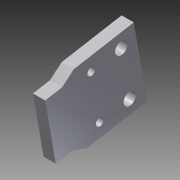
# Autodesk Inventor part: Arm_Link_1
Saved by Autodesk Inventor 2013 (Build 170138000, 138)
## iProperties
Created: 2014-05-15
Part Number: Arm_Link_1
Material: アセタール樹脂、白
Document SubType Name: Modeling
Designer: andou
Density: 1.425 g/cm^3
Mass: 3.20612 g
Surface Area: 16.6832 cm^2
Volume: 2.24991 cm^3
Author: andou
Autodesk Inventor part; units mm, degrees
ref_plane "YZ Plane" through (0, 0, 0) normal (1, 0, 0) x (0, 1, 0)
ref_plane "XZ Plane" through (0, 0, 0) normal (0, 1, 0) x (-1, 0, 0)
ref_plane "XY Plane" through (0, 0, 0) normal (0, 0, 1) x (1, 0, 0)
sketch "スケッチ2" plane through (0, 0, 0) normal (1, 0, 0) x (0, 1, 0)
  line L0 (0, 0) -> (-84.4498, 0)
  line L1 (-84.4498, -20) -> (1.7498, -20)
  line L2 (0, 0) -> (83.1668, 14.6646)
  line L3 (86.6398, -5.0316) -> (1.7498, -20)
  arc A0 (87.251, 14.537) -> (83.1668, 14.6646) centre (84.9033, 4.8165) ccw
  arc A1 (86.6398, -5.0316) -> (90.434, -3.5148) centre (84.9033, 4.8165) ccw
  arc A2 (-88.4498, -19.1652) -> (-84.4498, -20) centre (-84.4498, -10) ccw
  arc A3 (-84.4498, 0) -> (-88.4498, -0.8348) centre (-84.4498, -10) ccw
  arc A4 (-84.4498, -14) -> (-84.4498, -6) centre (-84.4498, -10) ccw
  line L4 (-84.4498, -6) -> (-88.4498, -6)
  line L5 (-84.4498, -14) -> (-88.4498, -14)
  line L6 (-88.4498, -0.8348) -> (-88.4498, -6)
  line L7 (-88.4498, -14) -> (-88.4498, -19.1652)
  line L8 (87.251, 14.537) -> (88.1479, 9.4503)
  line L9 (89.5371, 1.5718) -> (90.434, -3.5148)
  line L10 (1.7498, -20) -> (0, 0)
  line L11 (88.1479, 9.4503) -> (89.5371, 1.5718)
  dimension "d21" = 20
  dimension "d22" = 10
  dimension "d23" = 170
  dimension "d25" = 10
  dimension "d27" = 10
  dimension "d31" = 8
  dimension "d33" = 4
  dimension "d35" = 4
  dimension "d36" = 170
  constraints: 24 end point, 10 point on circle, 8 perpendicular, 5 centre point, 4 equal length, 3 equal radius, 2 parallel, 2 tangent, 1 coincident, 1 collinear, 1 horizontal
  measures "d21" distance between parallel lines of L0 L1
  measures "d22" distance from line of L0 A2.centre
  measures "d23" angle of L0 L2
  measures "d25" distance from line of L3 A0.centre
  measures "d27" radius of A3
  measures "d31" diameter of A4
  measures "d33" distance from line of L6 A2.centre
  measures "d35" distance from line of L8 L2.end
  measures "d36" distance of A2.centre A0.centre
extrude "押し出し1" add sketch "スケッチ2" along normal blind 4
sketch "スケッチ4" plane through (0, 0, 0) normal (-1, 0, 0) x (0, 0, 1)
  line L0 (-20, 1.7498) -> (-5.0316, 86.6398) projected
  line L1 (-20, -84.4498) -> (-20, 1.7498) projected
  circle A0 centre (-15, -8.7259) radius 1
  circle A1 centre (-13.2569, 11.198) radius 1
  line L2 (-15, -8.7259) -> (-13.2569, 11.198)
  dimension "d57" = 2
  dimension "d59" = 20
  dimension "d60" = 175
  dimension "d61" = 5
  dimension "d62" = 5
  constraints: 2 centre point, 2 end point, 1 equal radius
  measures "d57" diameter of A0
  measures "d59" distance of L2.start L2.end
  measures "d60" angle of L1 L2
  measures "d61" distance from line of L1 L2.start
  measures "d62" distance from line of L0 L2.end
hole "穴2" at (0, -8.7259, -15) at (0, 11.198, -13.2569) direction (1, 0, 0) diameter 1.6 end through all
sketch "スケッチ6" plane through (4, 0, 0) normal (1, 0, 0) x (0, 0, -1)
  line L0 (20, 1.7498) -> (5.0316, 86.6398) projected
  arc A0 (5.0316, 86.6398) -> (3.5148, 90.434) centre (-4.8165, 84.9033) ccw projected
  line L1 (3.5148, 90.434) -> (-14.537, 87.251) projected
  arc A1 (-14.537, 87.251) -> (-14.6646, 83.1668) centre (-4.8165, 84.9033) ccw projected
  line L2 (-14.6646, 83.1668) -> (0, 0) projected
  line L3 (-9.3978, 53.2975) -> (-12.6117, 57.1277)
  line L4 (-14.537, 87.251) -> (-17.8212, 86.6719)
  line L5 (-17.8212, 86.6719) -> (-12.6117, 57.1277)
  line L6 (3.5148, 90.434) -> (6.799, 91.0131)
  line L7 (6.799, 91.0131) -> (12.0085, 61.4689)
  line L8 (12.0085, 61.4689) -> (10.2984, 56.7704)
  dimension "d75" = 150
  dimension "d76" = 150
  dimension "d77" = 2.5
  dimension "d78" = 2.5
  dimension "d79" = 30
  constraints: 12 end point, 3 parallel, 2 collinear, 2 point on line
  measures "d75" angle of L2 L3
  measures "d76" angle of L0 L8
  measures "d77" distance between parallel lines of L0 L7
  measures "d78" distance between parallel lines of L2 L5
  measures "d79" distance of L4.end L3.end
extrude "押し出し2" add sketch "スケッチ6" against normal blind 4
sketch "スケッチ5" plane through (4, 0, 0) normal (1, 0, 0) x (0, 0, -1)
  line L0 (3.5148, 90.434) -> (-14.537, 87.251) projected
  line L1 (-14.6646, 83.1668) -> (0, 0) projected
  circle A0 centre (-10.7848, 72.6812) radius 1.5
  circle A1 centre (4.9721, 75.4596) radius 1.5
  line L2 (-12.6117, 57.1277) -> (-17.8212, 86.6719) projected
  line L3 (-17.8212, 86.6719) -> (6.799, 91.0131) projected
  line L4 (6.799, 91.0131) -> (12.0085, 61.4689) projected
  line L5 (12.0085, 61.4689) -> (10.2984, 56.7704) projected
  line L6 (10.2984, 56.7704) -> (20, 1.7498) projected
  line L7 (20, 1.7498) -> (20, -84.4498) projected
  arc A2 (19.1652, -88.4498) -> (20, -84.4498) centre (10, -84.4498) ccw projected
  line L8 (19.1652, -88.4498) -> (14, -88.4498) projected
  line L9 (14, -88.4498) -> (14, -84.4498) projected
  arc A3 (14, -84.4498) -> (6, -84.4498) centre (10, -84.4498) ccw projected
  line L10 (6, -84.4498) -> (6, -88.4498) projected
  line L11 (6, -88.4498) -> (0.8348, -88.4498) projected
  arc A4 (0, -84.4498) -> (0.8348, -88.4498) centre (10, -84.4498) ccw projected
  line L12 (0, -84.4498) -> (0, 0) projected
  line L13 (0, 0) -> (-9.3978, 53.2975) projected
  line L14 (-9.3978, 53.2975) -> (-12.6117, 57.1277) projected
  circle A5 centre (15, -8.7259) radius 0.8 projected
  circle A6 centre (13.2569, 11.198) radius 0.8 projected
  dimension "d70" = 15
  dimension "d71" = 15
  dimension "d72" = 3
  dimension "d73" = 16
  dimension "d74" = 2
  constraints: 2 centre point, 1 equal radius
  measures "d70" distance from line of L0 A0.centre
  measures "d71" distance from line of L0 A1.centre
  measures "d72" diameter of A1
  measures "d73" distance of A1.centre A0.centre
  measures "d74" distance from line of L1 A0.centre
hole "穴3" at (4, 72.6812, 10.7848) at (4, 75.4596, -4.9721) direction (-1, 0, 0) diameter 4 end through all
sketch "スケッチ7" plane through (4, 0, 0) normal (1, 0, 0) x (0, 0, -1)
  arc A0 (0, -84.4498) -> (0.8348, -88.4498) centre (10, -84.4498) ccw projected
  line L0 (0.8348, -88.4498) -> (6, -88.4498) projected
  circle A1 centre (3, -84.4498) radius 1
  dimension "d89" = 4
  dimension "d90" = 7
  dimension "d91" = 2
  constraints: 1 centre point
  measures "d89" distance from line of L0 A1.centre
  measures "d90" distance of A1.centre A0.centre
  measures "d91" diameter of A1
hole "穴4" at (4, -84.4498, -3) direction (-1, 0, 0) diameter 2 end through all
pattern_circular "円形状パターン3" count 5 over 180 about axis through (0, -84.4498, -10) along (-1, 0, 0) of "穴4"
sketch "スケッチ8" plane through (4, 0, 0) normal (1, 0, 0) x (0, 0, -1)
  circle A0 centre (-10.7848, 72.6812) radius 2 projected
  circle A1 centre (4.9721, 75.4596) radius 2 projected
  line L0 (10.2984, 56.7704) -> (12.0085, 61.4689) projected
  line L1 (12.0085, 61.4689) -> (6.799, 91.0131) projected
  line L2 (6.799, 91.0131) -> (-17.8212, 86.6719) projected
  line L3 (-17.8212, 86.6719) -> (-12.6117, 57.1277) projected
  line L4 (-12.6117, 57.1277) -> (-9.3978, 53.2975) projected
  line L5 (-9.3978, 53.2975) -> (0, 0) projected
  line L6 (20, 1.7498) -> (10.2984, 56.7704) projected
  line L7 (-8.4132, 47.7137) -> (11.2829, 51.1867)
  dimension "d122" = 40
  constraints: 2 end point, 2 point on line, 1 parallel, 1 perpendicular
  measures "d122" distance between parallel lines of L7 L2
extrude "押し出し3" cut sketch "スケッチ8" against normal blind 4 keep common part
sketch "スケッチ9" plane through (4, 0, 0) normal (1, 0, 0) x (0, 0, -1)
  line L0 (6.799, 91.0131) -> (-17.8212, 86.6719) projected
  line L1 (-17.8212, 86.6719) -> (-12.6117, 57.1277) projected
  circle A0 centre (-9.0483, 62.8332) radius 1.5
  circle A1 centre (6.7086, 65.6115) radius 1.5
  point P0 (0, 0)
  dimension "d104" = 16
  dimension "d106" = 3
  dimension "d107" = 4.5
  dimension "d110" = 25
  dimension "d111" = 25
  constraints: 2 centre point, 1 equal radius
  measures "d104" distance of A1.centre A0.centre
  measures "d106" diameter of A1
  measures "d107" distance from line of L1 A0.centre
  measures "d110" distance from line of L0 A0.centre
  measures "d111" distance from line of L0 A1.centre
hole "穴5" at (4, 62.8332, 9.0483) at (4, 65.6115, -6.7086) direction (-1, 0, 0) diameter 2.5 end through all
sketch "スケッチ10" plane through (4, 0, 0) normal (1, 0, 0) x (0, 0, -1)
  line L0 (12.0085, 61.4689) -> (6.799, 91.0131) projected
  line L1 (6.799, 91.0131) -> (-17.8212, 86.6719) projected
  line L2 (-17.8212, 86.6719) -> (-12.6117, 57.1277) projected
  line L3 (-16.0847, 76.8238) -> (8.5355, 81.1651)
  point P0 (0, 0)
  dimension "d119" = 10
  constraints: 2 end point, 2 point on line, 1 perpendicular
  measures "d119" distance between parallel lines of L1 L3
extrude "押し出し4" cut sketch "スケッチ10" against normal blind 4
